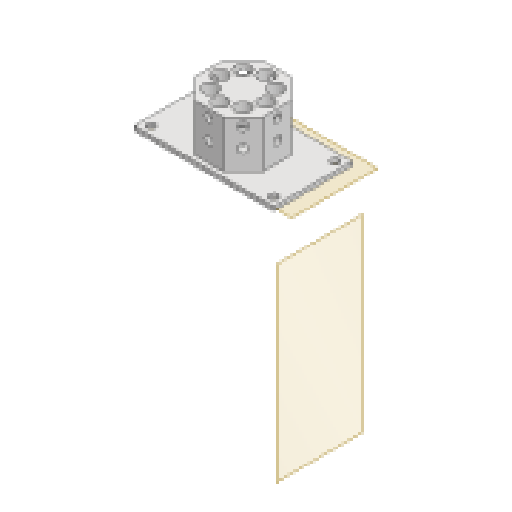
# Autodesk Inventor part: LED_holder_head_v1
Saved by Autodesk Inventor 2023 (Build 270158000, 158)
## iProperties
Created: 2022-09-24
Part Number: LED_holder_head_v1
Material: Generic
Document SubType Name: Modeling
Designer: CDT
Density: 1 g/cm^3
Appearance: Default
Author: CDT
Autodesk Inventor part; units mm, degrees
ref_plane "YZ Plane" through (0, 0, 0) normal (1, 0, 0) x (0, 1, 0)
ref_plane "XZ Plane" through (0, 0, 0) normal (0, 1, 0) x (-1, 0, 0)
ref_plane "XY Plane" through (0, 0, 0) normal (0, 0, 1) x (1, 0, 0)
ref_plane "Work Plane1" through (-109.5412, -279.6164, 416.6453) normal (1, 0, 0) x (0, 0.0002625, -1)
ref_plane "Work Plane2" through (-131.697, -198.1127, 402.6667) normal (0, 1, 0.0002625) x (-1, 0, 0)
sketch "Sketch1" plane through (-131.697, -198.1127, 402.6667) normal (0, 1, 0.0002625) x (-1, 0, 0)
  line L0 (27.8442, 16.4675) -> (-22.1558, 16.4675)
  line L1 (-22.1558, 16.4675) -> (-22.1558, -11.5325)
  line L2 (-22.1558, -11.5325) -> (27.8442, -11.5325)
  line L3 (27.8442, -11.5325) -> (27.8442, 16.4675)
  point P0 (-131.697, -402.7187)
  dimension "d0" = 28
  dimension "d1" = 50
  constraints: 8 end point, 2 parallel, 1 horizontal, 1 perpendicular
  measures "d0" distance between parallel lines of L2 L0
  measures "d1" distance between parallel lines of L1 L3
extrude "Extrusion1" add sketch "Sketch1" along normal blind 1.5
sketch "Sketch3" plane through (-131.697, -196.6127, 402.6671) normal (0, 1, 0.0002625) x (1, 0, 0)
  circle A0 centre (19.1558, -13.4675) radius 1.5
  circle A1 centre (-24.8442, -13.4675) radius 1.5
  circle A2 centre (19.1558, 8.5325) radius 1.5
  circle A3 centre (-24.8442, 8.5325) radius 1.5
  line L0 (-27.8442, 11.5325) -> (-27.8442, -16.4675) projected
  line L1 (-27.8442, -16.4675) -> (22.1558, -16.4675) projected
  line L2 (22.1558, -16.4675) -> (22.1558, 11.5325) projected
  line L3 (22.1558, 11.5325) -> (-27.8442, 11.5325) projected
  point P0 (131.697, 402.7187)
  dimension "d8" = 3
  dimension "d9" = 3
  dimension "d10" = 3
  dimension "d11" = 3
  dimension "d12" = 3
  dimension "d13" = 3
  dimension "d14" = 3
  dimension "d15" = 3
  dimension "d16" = 3
  dimension "d17" = 3
  dimension "d18" = 3
  dimension "d19" = 3
  constraints: 4 centre point
  measures "d8" diameter of A0
  measures "d9" diameter of A1
  measures "d10" diameter of A2
  measures "d11" diameter of A3
  measures "d12" distance from line of L0 A1.centre
  measures "d13" distance from line of L1 A1.centre
  measures "d14" distance from line of L1 A0.centre
  measures "d15" distance from line of L2 A0.centre
  measures "d16" distance from line of L2 A2.centre
  measures "d17" distance from line of L3 A2.centre
  measures "d18" distance from line of L3 A3.centre
  measures "d19" distance from line of L0 A3.centre
extrude "Extrusion2" cut sketch "Sketch3" against normal through all contours A0 | A1 | A2 | A3
sketch "Sketch4" plane through (-131.697, -196.6127, 402.6671) normal (0, 1, 0.0002625) x (1, 0, 0)
  line L0 (22.1558, -16.4675) -> (22.1558, 11.5325) projected
  line L1 (-27.8442, 11.5325) -> (-27.8442, -16.4675) projected
  line L2 (22.1558, 11.5325) -> (-27.8442, 11.5325) projected
  line L3 (-27.8442, -16.4675) -> (22.1558, -16.4675) projected
  line L4 (9.4058, 2.6067) -> (9.4058, -7.5416)
  line L5 (9.4058, -7.5416) -> (2.2299, -14.7175)
  line L6 (2.2299, -14.7175) -> (-7.9184, -14.7175)
  line L7 (-7.9184, -14.7175) -> (-15.0942, -7.5416)
  line L8 (-15.0942, -7.5416) -> (-15.0942, 2.6067)
  line L9 (-15.0942, 2.6067) -> (-7.9184, 9.7825)
  line L10 (-7.9184, 9.7825) -> (2.2299, 9.7825)
  line L11 (2.2299, 9.7825) -> (9.4058, 2.6067)
  point P0 (131.697, 402.7187)
  point P1 (-2.8442, -2.4675)
  dimension "d37" = 180
  dimension "d38" = 25
  dimension "d39" = 25
  dimension "d40" = 14
  dimension "d41" = 14
  dimension "d42" = 24.5
  dimension "d43" = 90
  constraints: 16 end point, 17 other
  measures "d37" angle of L0 L4
  measures "d38" distance from line of L0 point (-2.844, -2.467)
  measures "d39" distance from line of L1 point (-2.844, -2.467)
  measures "d40" distance from line of L2 point (-2.844, -2.467)
  measures "d41" distance from line of L3 point (-2.844, -2.467)
  measures "d42" distance between parallel lines of L4 L8
  measures "d43" angle of L0 L10
extrude "Extrusion3" add sketch "Sketch4" along normal blind 16 contours L4 L5 L6 L7 L8 L9 L10 L11
sketch "Sketch5" plane through (-131.697, -180.6127, 402.6713) normal (0, 1, 0.0002625) x (1, 0, 0)
  circle A0 centre (-2.8442, -10.7175) radius 2.65
  line L0 (-7.9184, -14.7175) -> (2.2299, -14.7175) projected
  point P0 (131.697, 402.7187)
  dimension "d46" = 5.3
  dimension "d47" = 4
  dimension "d48" = 5.0741
  dimension "d49" = 5.0741
  constraints: 1 centre point
  measures "d46" diameter of A0
  measures "d47" distance from line of L0 A0.centre
  measures "d48" horizontal distance of L0.end A0.centre
  measures "d49" horizontal distance of L0.start A0.centre
extrude "Extrusion4" cut sketch "Sketch5" against normal blind 6
sketch "Sketch6" plane through (-131.697, -180.6127, 402.6713) normal (0, 1, 0.0002625) x (1, 0, 0)
  circle A0 centre (-2.8442, -2.4675) radius 1.25
  line L0 (22.1558, 11.5325) -> (-27.8442, 11.5325) projected
  line L1 (-27.8442, -16.4675) -> (22.1558, -16.4675) projected
  line L2 (-27.8442, 11.5325) -> (-27.8442, -16.4675) projected
  line L3 (22.1558, -16.4675) -> (22.1558, 11.5325) projected
  point P0 (131.697, 402.7187)
  point P1 (-2.8442, 11.5325)
  dimension "d52" = 2.5
  dimension "d53" = 14
  dimension "d54" = 14
  dimension "d55" = 25
  dimension "d56" = 25
  constraints: 1 centre point, 1 midpoint
  measures "d52" diameter of A0
  measures "d53" distance of point (-2.844, 11.533) A0.centre
  measures "d54" distance from line of L1 A0.centre
  measures "d55" distance from line of L2 A0.centre
  measures "d56" distance from line of L3 A0.centre
extrude "Extrusion5" cut sketch "Sketch6" against normal through all contours A0
pattern_circular "Circular Pattern1" count 8 over 360 about axis through (-134.5412, -180.6134, 405.1388) along (0, -1, -0.0002625) of "Extrusion4"
sketch "Sketch7" plane through (-134.5412, -186.6112, 396.8872) normal (0, 1, 0.0002625) x (1, 0, 0)
  circle A0 centre (0, 0) radius 0.625
  point P0 (134.5412, 396.9362)
  dimension "d62" = 1.25
  constraints: 1 centre point
  measures "d62" diameter of A0
extrude "Extrusion6" cut sketch "Sketch7" against normal through all
pattern_circular "Circular Pattern2" count 8 over 360 about axis through (-134.5412, -180.6134, 405.1388) along (0, -1, -0.0002625) of "Extrusion6"
sketch "Sketch8" plane through (-129.4671, -196.6102, 392.8846) normal (0, 0.0002625, -1) x (-1, 0, 0)
  circle A0 centre (5.0741, 13) radius 1.5
  circle A1 centre (5.0741, 6) radius 1.5
  line L0 (0, 0) -> (0, 16) projected
  line L1 (10.1482, 0) -> (10.1482, 16) projected
  line L2 (0, 16) -> (10.1482, 16) projected
  point P0 (-129.4671, 196.5071)
  dimension "d68" = 3
  dimension "d69" = 3
  dimension "d70" = 5.0741
  dimension "d71" = 5.0741
  dimension "d72" = 5.0741
  dimension "d73" = 5.0741
  dimension "d74" = 3
  dimension "d76" = 7
  constraints: 2 centre point
  measures "d68" diameter of A0
  measures "d69" diameter of A1
  measures "d70" distance from line of L0 A0.centre
  measures "d71" distance from line of L0 A1.centre
  measures "d72" distance from line of L1 A0.centre
  measures "d73" distance from line of L1 A1.centre
  measures "d74" distance from line of L2 A0.centre
  measures "d76" distance of A1.centre A0.centre
extrude "Extrusion7" cut sketch "Sketch8" against normal blind 4.5
pattern_circular "Circular Pattern3" count 8 over 360 about axis through (-134.5412, -180.6134, 405.1388) along (0, -1, -0.0002625) of "Extrusion7"
chamfer "Chamfer1" distance 11.5 angle 45 1 edges at (-135.7912, -198.1134, 405.1342)
sketch "Sketch9" plane through (-131.697, -180.6127, 402.6713) normal (0, 1, 0.0002625) x (1, 0, 0)
  circle A0 centre (-2.8442, -2.4675) radius 2
  circle A1 centre (-2.8442, -2.4675) radius 1.25 projected
  point P0 (131.697, 402.7187)
  dimension "d85" = 0
  dimension "d86" = 0
  dimension "d87" = 4
  constraints: 1 centre point
  measures "d85" distance of A1.centre A0.centre
  measures "d86" distance of A1.centre A0.centre
  measures "d87" diameter of A0
extrude "Extrusion8" add sketch "Sketch9" against normal blind 2 contours A0 | A1
fillet "Fillet1" radius 1.5 8 edges at (-131.8912, -186.6132, 396.8872) (-126.8338, -186.6144, 401.1774) (-126.2912, -186.6161, 407.7872) (-130.5814, -186.6174, 412.8447) (-137.1912, -186.6176, 413.3872) (-142.2487, -186.6164, 409.097) (-142.7912, -186.6147, 402.4872) (-138.501, -186.6134, 397.4297)
equation "\"d38\" = d39"
equation "\"d40\" = d41"
equation "\"d48\" = d49"
equation "\"d53\" = d54"
equation "\"d55\" = d56"
equation "\"d70\" = d72"
equation "\"d71\" = d70"
body "Solid1"
